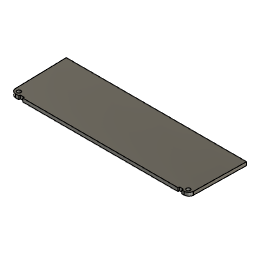
944 Immobiliser arduino mount v2 (Autodesk Fusion 360 design; units mm, degrees)
Autodesk Fusion 360 part; units mm, degrees
sketch "Sketch1" plane through (0, 0, 0) normal (0, 0, 1) x (1, 0, 0)
  line L0 (0, 60) -> (1.5, 0)
  line L1 (190.5, 60) -> (189.5, 0)
  line L2 (189.5, 0) -> (1.5, 0)
  line L3 (0, 60) -> (190.5, 60)
  constraint horizontal L2
  constraint parallel L2 L3
extrude "Extrude1" add sketch "Sketch1" along normal blind 3.5
fillet "Fillet1" radius 5 1 edges at (189.5, 0, 1.75)
fillet "Fillet2" radius 5 1 edges at (1.5, 0, 1.75)
sketch "Sketch2" plane through (0, 0, 0) normal (0, 0, 1) x (1, 0, 0)
sketch "Sketch3" plane through (0, 0, 3.5) normal (0, 0, 1) x (-1, 0, 0)
  arc A0 (-1.3781, -4.875) -> (-6.3766, 0) centre (-6.3766, -5) ccw
  line L0 (-6.3766, 0) -> (-184.5826, 0)
  arc A1 (-184.5826, 0) -> (-189.5819, -4.9167) centre (-184.5826, -5) ccw
  line L1 (-189.5819, -4.9167) -> (-190.5, -60)
  line L2 (-190.5, -60) -> (0, -60)
  line L3 (0, -60) -> (-1.3781, -4.875)
  circle A2 centre (-6, -4) radius 2
  circle A3 centre (-185, -4) radius 2
  dimension "d7" = 4
  dimension "d8" = 4
  measures "d7" diameter of A2
  measures "d8" diameter of A3
extrude "Extrude2" cut sketch "Sketch3" against normal blind 4 contours A2 | A3
sketch "Sketch4" plane through (0, 0, 3.5) normal (0, 0, 1) x (-1, 0, 0)
  circle A0 centre (-185, -4) radius 2
  circle A1 centre (-6, -4) radius 2
  arc A2 (-1.3781, -4.875) -> (-6.3766, 0) centre (-6.3766, -5) ccw
  line L0 (-6.3766, 0) -> (-184.5826, 0)
  arc A3 (-184.5826, 0) -> (-189.5819, -4.9167) centre (-184.5826, -5) ccw
  line L1 (-189.5819, -4.9167) -> (-190.5, -60)
  line L2 (-190.5, -60) -> (0, -60)
  line L3 (0, -60) -> (-1.3781, -4.875)
  line L4 (-10, -1.5) -> (-14, -1.5)
  line L5 (-14, -1.5) -> (-14, 0)
  line L6 (-14, 0) -> (-10, 0)
  line L7 (-10, 0) -> (-10, -1.5)
  constraint horizontal L4
  constraint vertical L5
  constraint horizontal L6
  constraint vertical L7
  constraint coincident L0 L5.end
extrude "Extrude3" cut sketch "Sketch4" against normal blind 4 contours L0 L4 L5 L6 L7
sketch "Sketch5" plane through (0, 0, 3.5) normal (0, 0, 1) x (-1, 0, 0)
  line L0 (-14, -1.5) -> (-14, 0)
  line L1 (-14, 0) -> (-184.5826, 0)
  arc A0 (-184.5826, 0) -> (-189.5819, -4.9167) centre (-184.5826, -5) ccw
  line L2 (-189.5819, -4.9167) -> (-190.5, -60)
  line L3 (-190.5, -60) -> (0, -60)
  line L4 (0, -60) -> (-1.3781, -4.875)
  arc A1 (-1.3781, -4.875) -> (-6.3766, 0) centre (-6.3766, -5) ccw
  line L5 (-6.3766, 0) -> (-10, 0)
  line L6 (-10, 0) -> (-10, -1.5)
  line L7 (-10, -1.5) -> (-14, -1.5)
  circle A2 centre (-185, -4) radius 2
  circle A3 centre (-6, -4) radius 2
  line L8 (-178, -1.5) -> (-182, -1.5)
  line L9 (-182, -1.5) -> (-182, 0)
  line L10 (-182, 0) -> (-178, 0)
  line L11 (-178, 0) -> (-178, -1.5)
  constraint horizontal L8
  constraint vertical L9
  constraint horizontal L10
  constraint vertical L11
  constraint coincident L1 L9.end
extrude "Extrude4" cut sketch "Sketch5" against normal blind 4 contours L1 L8 L9 L10 L11
